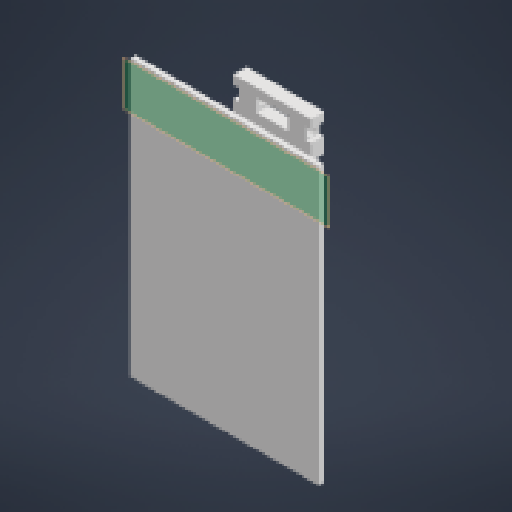
# Autodesk Inventor part: Head_Baseplate
Saved by Autodesk Inventor 2024 (Build 280153000, 153)
## iProperties
Created: 2025-09-25
Part Number: Head_Baseplate
Material: Generic
Document SubType Name: Modeling
Designer: kevin
Density: 1 g/cm^3
Appearance: Default
Author: kevin
Autodesk Inventor part; units mm, degrees
ref_plane "YZ Plane" through (0, 0, 0) normal (1, 0, 0) x (0, 1, 0)
ref_plane "XZ Plane" through (0, 0, 0) normal (0, 1, 0) x (-1, 0, 0)
ref_plane "XY Plane" through (0, 0, 0) normal (0, 0, 1) x (1, 0, 0)
sketch "Sketch1" plane through (0, 0, 0) normal (0, 0, 1) x (1, 0, 0)
  line L0 (51.9, 18.35) -> (51.9, 10.6) projected
  line L1 (72.1, 10.6) -> (72.1, 18.35) projected
  line L2 (51.9, 10.6) -> (72.1, 10.6) projected
  line L3 (51.9, 18.35) -> (72.1, 18.35) projected
  line L4 (0, 21.325) -> (0, 2)
  line L5 (124, 21.325) -> (124, 2)
  line L6 (51.5, 10.2) -> (51.5, 18.75)
  line L7 (51.5, 18.75) -> (72.5, 18.75)
  line L8 (72.5, 18.75) -> (72.5, 10.2)
  line L9 (72.5, 10.2) -> (51.5, 10.2)
  line L10 (51.5, 18.35) -> (39.7, 18.35)
  line L11 (39.7, 18.35) -> (39.7, 10.6)
  line L12 (39.7, 10.6) -> (51.5, 10.6)
  line L13 (62, 18.75) -> (62, 14.7524) construction
  line L14 (72.5, 18.35) -> (84.3, 18.35)
  line L15 (84.3, 18.35) -> (84.3, 10.6)
  line L16 (84.3, 10.6) -> (72.5, 10.6)
  line L17 (36.2904, 24.5) -> (87.7096, 24.5) projected
  line L18 (15.65, 0) -> (108.35, 0) projected
  line L19 (36.2904, 24.5) -> (87.7096, 24.5)
  line L20 (87.7096, 24.5) -> (87.7096, 0)
  line L21 (87.7096, 0) -> (36.2904, 0)
  line L22 (36.2904, 0) -> (36.2904, 24.5)
  line L23 (39.7, 18.35) -> (36.2904, 18.35)
  line L24 (39.7, 10.6) -> (36.2904, 10.6)
  line L25 (84.3, 10.6) -> (87.7096, 10.6)
  line L26 (84.3, 18.35) -> (87.7096, 18.35)
  point P0 (0, 0)
  dimension "d0" = 0.4
  dimension "d1" = 11.8
  constraints: 42 end point, 8 point on line, 6 perpendicular, 4 symmetric about line, 3 vertical, 2 horizontal, 2 parallel, 1 midpoint, 7 other
  measures "d0" distance between parallel lines of L0 L6
  measures "d1" distance of L10.start L10.end
extrude "Extrusion1" add sketch "Sketch1" along normal up to surface (8.8 mm away) contours L9 L8 L16 L25 L20 L18 L22 L24 L12 L6 | L12 L11 L10 L6 | L10 L23 L22 L17 L20 L26 L14 L8 L7 L6 | L8 L14 L15 L16
sketch "Sketch2" plane through (84.3, 10.6, 0) normal (1, 0, 0) x (0, 0, -1)
  circle A0 centre (-4.65, 3.875) radius 2.25 projected
  point P0 (0, -10.6)
extrude "Extrusion2" cut sketch "Sketch2" against normal up to surface (44.6 mm away)
sketch "Sketch3" plane through (84.3, 10.6, 0) normal (1, 0, 0) x (0, 0, -1)
  circle A0 centre (-4.65, 3.875) radius 2.25 projected
  circle A1 centre (-4.65, 3.875) radius 3.3
  point P0 (0, -10.6)
  dimension "d6" = 6.6
  constraints: 1 centre point, 1 coincident
  measures "d6" diameter of A1
extrude "Extrusion3" cut sketch "Sketch3" against normal blind 3.5 contours A0 | A1
sketch "Sketch4" plane through (39.7, 10.6, 0) normal (-1, 0, 0) x (0, 0, 1)
  circle A0 centre (4.65, 3.875) radius 2.25 projected
  circle A1 centre (4.65, 3.875) radius 3.3
  point P0 (0, -10.6)
  dimension "d9" = 6.6
  constraints: 1 centre point, 1 coincident
  measures "d9" diameter of A1
extrude "Extrusion4" cut sketch "Sketch4" against normal blind 3.5 contours A0 | A1
fillet "Fillet1" radius 1 4 edges at (51.5, 14.475, 0) (72.5, 14.475, 0) (62, 18.75, 0) (62, 10.2, 0)
ref_plane "Work Plane1" through (62, 0, 39.141) normal (0, 0, -1) x (-1, 0, 0)
body "Solid1"
